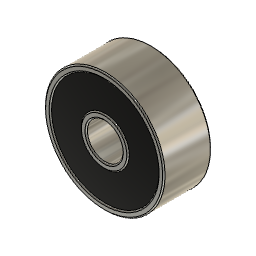
Full Prototype Build with Membrane Wings (Autodesk Fusion 360 archive; units mm, degrees)
design "Bearing 10 03"
Autodesk Fusion 360 part; units mm, degrees
note: some values were not read from the file. Chosen so that the rebuilt part matches the saved one: which face or edge a step refers to. Set by a fixed rule: which sketch regions a step uses.
sketch "Sketch1" plane through (0, 0, 0) normal (0, 1, 0) x (1, 0, 0)
  circle A0 centre (0, 0) radius 5
  circle A1 centre (0, 0) radius 1.5
  circle A2 centre (0, 0) radius 2
  circle A3 centre (0, 0) radius 4.5
  dimension "d1" = 10
  dimension "d2" = 3
  dimension "d3" = 4
  dimension "d4" = 9
  constraint coincident A0.centre A1.centre
  constraint concentric A0 A3
  measures "d1" diameter of A0
  measures "d2" diameter of A1
  measures "d3" diameter of A2
  measures "d4" diameter of A3
extrude "Extrude1" add sketch "Sketch1" along normal mid plane 4 makes body 1 at (1.9975, 1.3333, 0.0997) makes body 2 at (4.9938, 1.3333, 0.2492)
extrude "Extrude2" add sketch "Sketch1" along normal mid plane 3.8 separate body contours A3 makes body 3
fillet "Fillet1" radius 0.1 4 edges at (-4.6616, -2, -1.8081) (-4.6616, 2, 1.8081) (-4.1955, -2, 1.6273) (-4.1955, 2, -1.6273) on bodies 2
fillet "Fillet2" radius 0.1 4 edges at (-1.3985, 2, -0.5424) (-1.8647, 2, 0.7232) (-1.3985, -2, 0.5424) (-1.8647, -2, -0.7232) on bodies 1
equation "d7 = 2 mm - 0.1 mm"

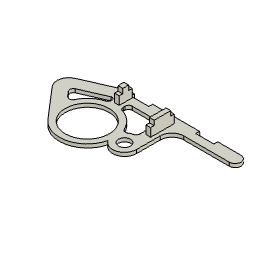
design "bottom_chassis"
Autodesk Fusion 360 part; units mm, degrees
sketch "Sketch1" plane through (0, 0, 0) normal (0, 0, 1) x (1, 0, 0)
  circle A0 centre (0, 0) radius 18.6
  line L0 (-40.1145, 10.4906) -> (-17.9049, -15.3744)
  line L1 (5, 25.3685) -> (5, 26.9321)
  line L2 (-5, 26.019) -> (-5, 25.3685)
  line L3 (-5, 40) -> (-36.5447, 26.1628)
  line L4 (-28.8171, 18.6328) -> (-7.8034, 27.8505)
  line L5 (-29.888, 13.9311) -> (-26.2116, 9.6495)
  arc A1 (-36.5447, 26.1628) -> (-40.1145, 10.4906) centre (-32.5276, 17.0051) ccw
  line L6 (15.2, 40) -> (15.2, 36.8)
  line L7 (15.2, 36.8) -> (0, 36.8)
  line L8 (0, 36.8) -> (0, 40)
  line L9 (15.2, 40) -> (55, 40)
  line L10 (70.2, 40) -> (70.2, 36.8)
  line L11 (70.2, 36.8) -> (55, 36.8)
  line L12 (55, 36.8) -> (55, 40)
  line L13 (-5, 40) -> (0, 40)
  line L14 (41.6, 0) -> (41.6, 20)
  arc A2 (90, 30) -> (90, 40) centre (90, 35) ccw
  line L15 (90, 30) -> (51.6, 30)
  line L16 (8, 29.9321) -> (28.6, 29.9321)
  line L17 (31.6, 26.9321) -> (31.6, 12.775)
  arc A3 (-17.9049, -15.3744) -> (22.9714, -5.4105) centre (0, 0) ccw
  arc A4 (21.5214, 9.6845) -> (7.0977, 22.5074) centre (0, 0) ccw
  arc A5 (-7.0977, 22.5074) -> (-21.236, 10.2952) centre (0, 0) ccw
  arc A6 (22.9714, -5.4105) -> (41.6, 0) centre (31.5, 0) ccw
  arc A7 (29.2641, 9.8494) -> (25.9158, 8.4159) centre (31.5, 0) ccw
  arc A8 (-28.8171, 18.6328) -> (-29.888, 13.9311) centre (-27.612, 15.8855) ccw
  arc A9 (-26.2116, 9.6495) -> (-21.236, 10.2952) centre (-23.9355, 11.6039) ccw
  arc A10 (-7.0977, 22.5074) -> (-5, 25.3685) centre (-8, 25.3685) ccw
  arc A11 (-5, 26.019) -> (-7.8034, 27.8505) centre (-7, 26.019) ccw
  arc A12 (8, 29.9321) -> (5, 26.9321) centre (8, 26.9321) ccw
  arc A13 (5, 25.3685) -> (7.0977, 22.5074) centre (8, 25.3685) ccw
  arc A14 (21.5214, 9.6845) -> (25.9158, 8.4159) centre (24.2571, 10.9156) ccw
  arc A15 (29.2641, 9.8494) -> (31.6, 12.775) centre (28.6, 12.775) ccw
  arc A16 (31.6, 26.9321) -> (28.6, 29.9321) centre (28.6, 26.9321) ccw
  arc A17 (51.6, 30) -> (41.6, 20) centre (51.6, 20) ccw
  line L18 (0, 40) -> (-5, 40)
  line L19 (90, 40) -> (70.2, 40)
  line L20 (55, 40) -> (15.2, 40)
  line L21 (-2, 36) -> (2, 36)
  line L22 (2, 36) -> (2, 25)
  line L23 (2, 25) -> (-2, 25)
  line L24 (-2, 25) -> (-2, 36)
  line L25 (-2, 33) -> (2, 33)
  line L26 (2, 33) -> (2, 28)
  line L27 (2, 28) -> (-2, 28)
  line L28 (-2, 28) -> (-2, 33)
  line L29 (34.6, 35) -> (38.6, 35)
  line L30 (38.6, 35) -> (38.6, 15)
  line L31 (38.6, 15) -> (34.6, 15)
  line L32 (34.6, 15) -> (34.6, 35)
  line L33 (34.6, 32) -> (38.6, 32)
  line L34 (34.6, 18) -> (38.6, 18)
  circle A18 centre (31.5, 0) radius 5.1
  dimension "d4" = 37.2
  dimension "d6" = 47.2
  dimension "d7" = 20.2
  dimension "d8" = 20
  dimension "d11" = 31.5
  dimension "d12" = 15.2
  dimension "d13" = 3.2
  dimension "d14" = 55
  dimension "d15" = 15.2
  dimension "d16" = 3.2
  dimension "d19" = 3
  dimension "d20" = 2
  dimension "d21" = 3
  dimension "d22" = 10
  dimension "d26" = 4
  dimension "d27" = 20
  dimension "d35" = 10.2
  constraint coincident A0.centre A3.centre
  constraint coincident L0.end A4
  constraint tangent L0 A4
  constraint tangent L0 A1
  constraint parallel L0 L5
  constraint tangent L3 A1
  constraint vertical L6
  constraint horizontal L7
  constraint vertical L8
  constraint perpendicular L6 L9
  constraint vertical L10
  constraint horizontal L11
  constraint vertical L12
  constraint tangent L14 A6
  constraint perpendicular L9 L14
  constraint tangent A2 L19
  constraint tangent A2 L15
  constraint perpendicular L14 L15
  constraint concentric A3 A4
  constraint concentric A4 A5
  constraint concentric A6 A7
  constraint tangent L4 A8
  constraint tangent L5 A8
  constraint tangent L5 A9
  constraint tangent A5 A9
  constraint equal A8 A9
  constraint tangent L2 A10
  constraint tangent A5 A10
  constraint equal A8 A10
  constraint tangent L4 A11
  constraint tangent L2 A11
  constraint tangent L16 A12
  constraint tangent L1 A12
  constraint tangent L1 A13
  constraint tangent A4 A13
  constraint equal A12 A13
  constraint tangent A4 A14
  constraint tangent A7 A14
  constraint equal A12 A14
  constraint tangent L17 A15
  constraint tangent A7 A15
  constraint equal A12 A15
  constraint tangent L16 A16
  constraint tangent L17 A16
  constraint equal A12 A16
  constraint tangent L15 A17
  constraint tangent L14 A17
  constraint collinear L18 L19
  constraint collinear L19 L20
  constraint horizontal L21
  constraint vertical L22
  constraint horizontal L23
  constraint vertical L24
  constraint horizontal L25
  constraint vertical L26
  constraint horizontal L27
  constraint vertical L28
  constraint coincident L22 L26.end
  constraint coincident L24 L25.start
  constraint horizontal L29
  constraint vertical L30
  constraint horizontal L31
  constraint vertical L32
  constraint perpendicular L32 L33
  constraint perpendicular L32 L34
  constraint coincident L30 L34.end
  constraint coincident L32 L34.start
  constraint coincident L32 L33.start
  constraint coincident L30 L33.end
  constraint concentric A6 A18
  measures "d4" diameter of A0
  measures "d6" diameter of A4
  measures "d7" diameter of A6
  measures "d8" diameter of A1
  measures "d11" distance of A0.centre A6.centre
  measures "d12" distance of L8.end L6.start
  measures "d13" distance of L8.end L7.end
  measures "d14" distance of L8.end L9.end
  measures "d15" distance of L9.end L10.start
  measures "d16" distance of L9.end L11.end
  measures "d19" radius of A8
  measures "d20" radius of A11
  measures "d21" radius of A12
  measures "d22" radius of A17
  measures "d26" distance of L29.start L29.end
  measures "d27" distance of L29.start L31.end
  measures "d35" diameter of A18
extrude "Extrude1" add sketch "Sketch1" against normal blind 4 contours L0 L3 A1 L6 L7 L8 L9 L10 L11 L12 L13 L14 A2 L15 A3 A6 A17 L18 L19 L20 | L21 L22 L24 L25 | L22 L24 L25 L26 L27 L28 | L22 L23 L24 L27 | L29 L30 L32 L33 | L30 L32 L33 L34 | L30 L31 L32 L34 | A18
extrude "Extrude2" add sketch "Sketch1" along normal blind 7 contours L21 L22 L24 L25 | L22 L23 L24 L27 | L29 L30 L32 L33 | L30 L31 L32 L34
extrude "Extrude3" add sketch "Sketch1" along normal blind 11 contours L22 L24 L25 L26 L27 L28 | L30 L32 L33 L34
extrude "Extrude4" cut sketch "Sketch1" against normal blind 10 contours A18
extrude "Extrude5" cut 1 faces at (33.2151, 36.6035, -4) along direction (0, 0, 1) blind 1
equation "d6 = 37.200 mm + 5 mm + 5 mm"
equation "d7 = 10.200 mm + 10 mm"
equation "d33 = 7 mm + 4 mm"

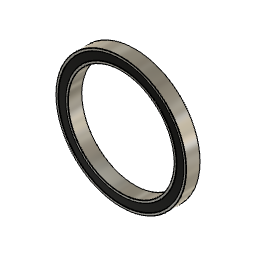
design "Bearing 37 30"
Autodesk Fusion 360 part; units mm, degrees
sketch "Sketch1" plane through (0, 0, 0) normal (0, 1, 0) x (1, 0, 0)
  circle A0 centre (0, 0) radius 15
  circle A1 centre (0, 0) radius 18.5
  circle A2 centre (0, 0) radius 15.75
  circle A3 centre (0, 0) radius 17.75
  dimension "d1" = 30
  dimension "d2" = 37
  dimension "d3" = 31.5
  dimension "d4" = 35.5
  constraint coincident A0.centre A1.centre
  constraint concentric A0 A2
  constraint concentric A2 A3
  measures "d1" diameter of A0
  measures "d2" diameter of A1
  measures "d3" diameter of A2
  measures "d4" diameter of A3
extrude "Extrude1" add sketch "Sketch1" along normal mid plane 4 makes body 1 at (15.7304, 1.3333, 0.7851) makes body 2 at (18.477, 1.3333, 0.9221)
extrude "Extrude2" add sketch "Sketch1" along normal mid plane 3.8 separate body contours A3 makes body 3
fillet "Fillet1" radius 0.1 8 edges at (-14.6842, -2, -5.6954) (-13.9849, -2, 5.4242) (-14.6842, 2, 5.6954) (-13.9849, 2, -5.4242) (-17.2481, -2, -6.6899) (-16.5488, -2, 6.4187) (-17.2481, 2, 6.6899) (-16.5488, 2, -6.4187) on bodies 1 2
equation "d7 = 2 mm - 0.1 mm"
